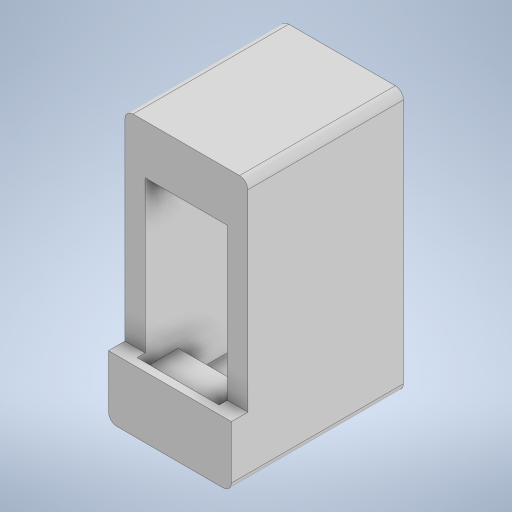
# Autodesk Inventor part: wirst
Saved by Autodesk Inventor 2023 (Build 270158000, 158)
## iProperties
Created: 2024-06-26
Part Number: wirst
Material: Generic
Document SubType Name: Modeling
Designer: Swoby
Density: 1 g/cm^3
Appearance: Default
Author: Swoby
Autodesk Inventor part; units mm, degrees
ref_plane "YZ Plane" through (0, 0, 0) normal (1, 0, 0) x (0, 1, 0)
ref_plane "XZ Plane" through (0, 0, 0) normal (0, 1, 0) x (-1, 0, 0)
ref_plane "XY Plane" through (0, 0, 0) normal (0, 0, 1) x (1, 0, 0)
sketch "Sketch1" plane through (0, 0, 0) normal (0, 0, 1) x (1, 0, 0)
  line L0 (-10, 18) -> (10, 18)
  line L1 (10, 18) -> (10, -36)
  line L2 (10, -36) -> (-10, -36)
  line L3 (-10, -36) -> (-10, 18)
  line L4 (-33.75, 0) -> (47.25, 0) construction
  line L5 (0, 28.5476) -> (0, -28.5476) construction
  line L6 (-13, 23) -> (13, 23)
  line L7 (15, 21) -> (15, -39)
  line L8 (13, -41) -> (-13, -41)
  line L9 (-15, -39) -> (-15, 21)
  arc A0 (-13, 23) -> (-15, 21) centre (-13, 21) ccw
  arc A1 (-15, -39) -> (-13, -41) centre (-13, -39) ccw
  arc A2 (13, -41) -> (15, -39) centre (13, -39) ccw
  arc A3 (15, 21) -> (13, 23) centre (13, 21) ccw
  point P0 (0, 0)
  dimension "d0" = 54
  dimension "d1" = 20
  dimension "d2" = 10
  dimension "d3" = 36
  dimension "d4" = 5
  dimension "d5" = 2
  constraints: 20 end point, 8 point on circle, 8 tangent, 4 centre point, 4 parallel, 3 equal radius, 2 horizontal, 2 perpendicular, 1 midpoint, 1 point on line, 1 vertical, 3 other
  measures "d0" distance of L0.end L1.end
  measures "d1" distance of L0.start L0.end
  measures "d2" distance between parallel lines of L3 L5
  measures "d3" distance from line of L2 point (0, 0)
  measures "d4" distance between parallel lines of L3 L9
  measures "d5" radius of A0
extrude "Extrusion1" add sketch "Sketch1" against normal blind 38
sketch "Sketch2" plane through (0, 0, 0) normal (0, 0, 1) x (1, 0, 0)
  line L0 (10, 18) -> (-10, 18) projected
  line L1 (-10, 18) -> (10, 18)
  line L2 (10, 18) -> (10, 11)
  line L3 (10, 11) -> (-10, 11)
  line L4 (-10, 11) -> (-10, 18)
  line L5 (10, 18) -> (10, -36) projected
  line L6 (10, -36) -> (-10, -36)
  line L7 (-10, -36) -> (-10, -29)
  line L8 (-10, -29) -> (10, -29)
  line L9 (10, -29) -> (10, -36)
  point P0 (0, 0)
  dimension "d8" = 7
  dimension "d9" = 7
  constraints: 16 end point, 4 parallel, 2 horizontal, 2 perpendicular, 1 point on line
  measures "d8" distance of L3.end L0.end
  measures "d9" distance of L6.end L7.end
extrude "Extrusion2" add sketch "Sketch2" against normal blind 8
sketch "Sketch3" plane through (0, 0, 0) normal (0, 0, 1) x (1, 0, 0)
  line L0 (-13, -41) -> (13, -41) projected
  arc A0 (13, -41) -> (15, -39) centre (13, -39) ccw projected
  line L1 (15, -39) -> (15, 21) projected
  arc A1 (15, 21) -> (13, 23) centre (13, 21) ccw projected
  line L2 (13, 23) -> (-13, 23) projected
  arc A2 (-13, 23) -> (-15, 21) centre (-13, 21) ccw projected
  line L3 (-15, 21) -> (-15, -39) projected
  arc A3 (-15, -39) -> (-13, -41) centre (-13, -39) ccw projected
  line L4 (10, 11) -> (10, -29) projected
  line L5 (10, -29) -> (-10, -29) projected
  line L6 (-10, -29) -> (-10, 11) projected
  line L7 (-10, 11) -> (10, 11) projected
  line L8 (-15, -26) -> (-10, -26)
  line L9 (10, -36) -> (10, 18) projected
  line L10 (10, -26) -> (15, -26)
  point P0 (0, 0)
  point P1 (10, -26)
  dimension "d12" = 15
  constraints: 6 point on line, 4 end point, 1 perpendicular
  measures "d12" distance between parallel lines of L0 L8
extrude "Extrusion3" add sketch "Sketch3" along normal blind 2 contours A3 L3 L8 L6 L5 L4 L10 L1 A0 L0
sketch "Sketch4" plane through (0, 0, 2) normal (0, 0, 1) x (1, 0, 0)
  line L0 (15, -39) -> (15, -26) projected
  line L1 (15, -26) -> (10, -26) projected
  line L2 (10, -26) -> (10, -29) projected
  line L3 (10, -29) -> (-10, -29) projected
  line L4 (-10, -29) -> (-10, -26) projected
  line L5 (-10, -26) -> (-15, -26) projected
  line L6 (-15, -26) -> (-15, -39) projected
  arc A0 (-15, -39) -> (-13, -41) centre (-13, -39) ccw projected
  line L7 (-13, -41) -> (13, -41) projected
  arc A1 (13, -41) -> (15, -39) centre (13, -39) ccw projected
  line L8 (-10, -26) -> (10, -26)
  point P0 (0, 0)
  constraints: 2 end point, 1 perpendicular
extrude "Extrusion4" add sketch "Sketch4" along normal blind 2
body "Solid1"
